Autodesk Fusion 360 part; units mm, degrees
(part 2 of 3)
sketch "Pocket SRL sketch" plane through (0, 0, 0) normal (0, 0, 1) x (1, 0, 0) in component "Upper frame"
  line L0 (-81.4, 57.15) -> (-81.4, 62.85)
  line L1 (-81.4, 62.85) -> (-62.2, 62.85)
  line L2 (-62.2, 62.85) -> (-62.2, 57.15)
  line L3 (-62.2, 57.15) -> (-81.4, 57.15)
extrude "Pocket SRL" cut sketch "Pocket SRL sketch" along normal blind 24 from surface at 89 bodies 27 in component "Upper frame"
sketch "Beam SRL sketch" plane through (0, 0, 0) normal (0, 0, 1) x (1, 0, 0) in component "Upper frame"
  line L0 (-80.8, 60) -> (-80.8, 80.6769)
  line L1 (-80.8, 80.6769) -> (-62.8, 80.6769)
  line L2 (-62.8, 80.6769) -> (-62.8, 60)
  line L3 (-62.8, 60) -> (-80.8, 60)
extrude "Beam SRL" cut sketch "Beam SRL sketch" along normal blind 18 from surface at 91 bodies 27 in component "Upper frame"
sketch "Pocket SRR sketch" plane through (0, 0, 0) normal (0, 0, 1) x (1, 0, 0) in component "Upper frame"
  line L0 (-62.2, -57.15) -> (-62.2, -62.85)
  line L1 (-62.2, -62.85) -> (-81.4, -62.85)
  line L2 (-81.4, -62.85) -> (-81.4, -57.15)
  line L3 (-81.4, -57.15) -> (-62.2, -57.15)
extrude "Pocket SRR" cut sketch "Pocket SRR sketch" along normal blind 24 from surface at 89 bodies 27 in component "Upper frame"
sketch "Beam SRR sketch" plane through (0, 0, 0) normal (0, 0, 1) x (1, 0, 0) in component "Upper frame"
  line L0 (-62.8, -60) -> (-62.8, -80.6769)
  line L1 (-62.8, -80.6769) -> (-80.8, -80.6769)
  line L2 (-80.8, -80.6769) -> (-80.8, -60)
  line L3 (-80.8, -60) -> (-62.8, -60)
extrude "Beam SRR" cut sketch "Beam SRR sketch" along normal blind 18 from surface at 91 bodies 27 in component "Upper frame"
sketch "Pocket RL sketch" plane through (0, 0, 0) normal (0, 0, 1) x (1, 0, 0) in component "Upper frame"
  line L0 (-81.15, 35.4) -> (-86.85, 35.4)
  line L1 (-86.85, 35.4) -> (-86.85, 54.6)
  line L2 (-86.85, 54.6) -> (-81.15, 54.6)
  line L3 (-81.15, 54.6) -> (-81.15, 35.4)
extrude "Pocket RL" cut sketch "Pocket RL sketch" along normal blind 24 from surface at 89 bodies 27 in component "Upper frame"
sketch "Beam RL sketch" plane through (0, 0, 0) normal (0, 0, 1) x (1, 0, 0) in component "Upper frame"
  line L0 (-84, 36) -> (-98.1784, 36)
  line L1 (-98.1784, 36) -> (-98.1784, 54)
  line L2 (-98.1784, 54) -> (-84, 54)
  line L3 (-84, 54) -> (-84, 36)
extrude "Beam RL" cut sketch "Beam RL sketch" along normal blind 18 from surface at 91 bodies 27 in component "Upper frame"
sketch "Pocket RR sketch" plane through (0, 0, 0) normal (0, 0, 1) x (1, 0, 0) in component "Upper frame"
  line L0 (-81.15, -54.6) -> (-86.85, -54.6)
  line L1 (-86.85, -54.6) -> (-86.85, -35.4)
  line L2 (-86.85, -35.4) -> (-81.15, -35.4)
  line L3 (-81.15, -35.4) -> (-81.15, -54.6)
extrude "Pocket RR" cut sketch "Pocket RR sketch" along normal blind 24 from surface at 89 bodies 27 in component "Upper frame"
sketch "Beam RR sketch" plane through (0, 0, 0) normal (0, 0, 1) x (1, 0, 0) in component "Upper frame"
  line L0 (-84, -54) -> (-98.1784, -54)
  line L1 (-98.1784, -54) -> (-98.1784, -36)
  line L2 (-98.1784, -36) -> (-84, -36)
  line L3 (-84, -36) -> (-84, -54)
extrude "Beam RR" cut sketch "Beam RR sketch" along normal blind 18 from surface at 91 bodies 27 in component "Upper frame"
sketch "Camera window L sketch" plane through (0, 0, 0) normal (0, 1, 0) x (1, 0, 0) in component "Upper frame"
  line L0 (-10.9288, -86) -> (17.0712, -86)
  line L1 (17.0712, -86) -> (17.0712, -106)
  line L2 (17.0712, -106) -> (-10.9288, -106)
  line L3 (-10.9288, -106) -> (-10.9288, -86)
extrude "Camera window L" cut sketch "Camera window L sketch" along normal blind 24 from surface at 84 bodies 27 in component "Upper frame"
sketch "Camera window R sketch" plane through (0, 0, 0) normal (0, 1, 0) x (1, 0, 0) in component "Upper frame"
  line L0 (-10.9288, -86) -> (17.0712, -86)
  line L1 (17.0712, -86) -> (17.0712, -106)
  line L2 (17.0712, -106) -> (-10.9288, -106)
  line L3 (-10.9288, -106) -> (-10.9288, -86)
extrude "Camera window R" cut sketch "Camera window R sketch" along normal blind 24 from surface at -108 bodies 27 in component "Upper frame"
sketch "VL53L0X module F sketch" plane through (0, 0, 0) normal (0, 0, 1) x (1, 0, 0) in component "ToF F"
  line L0 (92.75, -9) -> (97.25, -9)
  line L1 (97.25, -9) -> (97.25, 9)
  line L2 (97.25, 9) -> (92.75, 9)
  line L3 (92.75, 9) -> (92.75, -9)
extrude "VL53L0X module F" add sketch "VL53L0X module F sketch" along normal blind 21 from surface at 89.5 separate body makes body 28 in component "ToF F"
sketch "VL53L0X chip F sketch" plane through (0, 0, 0) normal (0, 0, 1) x (1, 0, 0) in component "ToF F"
  line L0 (97.25, -2.2) -> (98.25, -2.2)
  line L1 (98.25, -2.2) -> (98.25, 2.2)
  line L2 (98.25, 2.2) -> (97.25, 2.2)
  line L3 (97.25, 2.2) -> (97.25, -2.2)
extrude "VL53L0X chip F" add sketch "VL53L0X chip F sketch" along normal blind 2.4 from surface at 98.8 separate body makes body 29 in component "ToF F"
sketch "VL53L0X module FL sketch" plane through (0, 0, 0) normal (0, 0, 1) x (1, 0, 0) in component "ToF FL"
  line L0 (91.4888, 32.7315) -> (95.5672, 34.6333)
  line L1 (95.5672, 34.6333) -> (87.9601, 50.9469)
  line L2 (87.9601, 50.9469) -> (83.8817, 49.0451)
  line L3 (83.8817, 49.0451) -> (91.4888, 32.7315)
extrude "VL53L0X module FL" add sketch "VL53L0X module FL sketch" along normal blind 21 from surface at 89.5 separate body makes body 30 in component "ToF FL"
sketch "VL53L0X chip FL sketch" plane through (0, 0, 0) normal (0, 0, 1) x (1, 0, 0) in component "ToF FL"
  line L0 (92.6934, 40.7962) -> (93.5997, 41.2188)
  line L1 (93.5997, 41.2188) -> (91.7402, 45.2066)
  line L2 (91.7402, 45.2066) -> (90.8339, 44.784)
  line L3 (90.8339, 44.784) -> (92.6934, 40.7962)
extrude "VL53L0X chip FL" add sketch "VL53L0X chip FL sketch" along normal blind 2.4 from surface at 98.8 separate body makes body 31 in component "ToF FL"
sketch "VL53L0X module FR sketch" plane through (0, 0, 0) normal (0, 0, 1) x (1, 0, 0) in component "ToF FR"
  line L0 (83.8817, -49.0451) -> (87.9601, -50.9469)
  line L1 (87.9601, -50.9469) -> (95.5672, -34.6333)
  line L2 (95.5672, -34.6333) -> (91.4888, -32.7315)
  line L3 (91.4888, -32.7315) -> (83.8817, -49.0451)
extrude "VL53L0X module FR" add sketch "VL53L0X module FR sketch" along normal blind 21 from surface at 89.5 separate body makes body 32 in component "ToF FR"
sketch "VL53L0X chip FR sketch" plane through (0, 0, 0) normal (0, 0, 1) x (1, 0, 0) in component "ToF FR"
  line L0 (90.8339, -44.784) -> (91.7402, -45.2066)
  line L1 (91.7402, -45.2066) -> (93.5997, -41.2188)
  line L2 (93.5997, -41.2188) -> (92.6934, -40.7962)
  line L3 (92.6934, -40.7962) -> (90.8339, -44.784)
extrude "VL53L0X chip FR" add sketch "VL53L0X chip FR sketch" along normal blind 2.4 from surface at 98.8 separate body makes body 33 in component "ToF FR"
sketch "VL53L0X module SFL sketch" plane through (0, 0, 0) normal (0, 0, 1) x (1, 0, 0) in component "ToF SFL"
  line L0 (80.8, 57.75) -> (80.8, 62.25)
  line L1 (80.8, 62.25) -> (62.8, 62.25)
  line L2 (62.8, 62.25) -> (62.8, 57.75)
  line L3 (62.8, 57.75) -> (80.8, 57.75)
extrude "VL53L0X module SFL" add sketch "VL53L0X module SFL sketch" along normal blind 21 from surface at 89.5 separate body makes body 34 in component "ToF SFL"
sketch "VL53L0X chip SFL sketch" plane through (0, 0, 0) normal (0, 0, 1) x (1, 0, 0) in component "ToF SFL"
  line L0 (74, 62.25) -> (74, 63.25)
  line L1 (74, 63.25) -> (69.6, 63.25)
  line L2 (69.6, 63.25) -> (69.6, 62.25)
  line L3 (69.6, 62.25) -> (74, 62.25)
extrude "VL53L0X chip SFL" add sketch "VL53L0X chip SFL sketch" along normal blind 2.4 from surface at 98.8 separate body makes body 35 in component "ToF SFL"
sketch "VL53L0X module SFR sketch" plane through (0, 0, 0) normal (0, 0, 1) x (1, 0, 0) in component "ToF SFR"
  line L0 (62.8, -57.75) -> (62.8, -62.25)
  line L1 (62.8, -62.25) -> (80.8, -62.25)
  line L2 (80.8, -62.25) -> (80.8, -57.75)
  line L3 (80.8, -57.75) -> (62.8, -57.75)
extrude "VL53L0X module SFR" add sketch "VL53L0X module SFR sketch" along normal blind 21 from surface at 89.5 separate body makes body 36 in component "ToF SFR"
sketch "VL53L0X chip SFR sketch" plane through (0, 0, 0) normal (0, 0, 1) x (1, 0, 0) in component "ToF SFR"
  line L0 (69.6, -62.25) -> (69.6, -63.25)
  line L1 (69.6, -63.25) -> (74, -63.25)
  line L2 (74, -63.25) -> (74, -62.25)
  line L3 (74, -62.25) -> (69.6, -62.25)
extrude "VL53L0X chip SFR" add sketch "VL53L0X chip SFR sketch" along normal blind 2.4 from surface at 98.8 separate body makes body 37 in component "ToF SFR"
sketch "VL53L0X module SRL sketch" plane through (0, 0, 0) normal (0, 0, 1) x (1, 0, 0) in component "ToF SRL"
  line L0 (-62.8, 57.75) -> (-62.8, 62.25)
  line L1 (-62.8, 62.25) -> (-80.8, 62.25)
  line L2 (-80.8, 62.25) -> (-80.8, 57.75)
  line L3 (-80.8, 57.75) -> (-62.8, 57.75)
extrude "VL53L0X module SRL" add sketch "VL53L0X module SRL sketch" along normal blind 21 from surface at 89.5 separate body makes body 38 in component "ToF SRL"
sketch "VL53L0X chip SRL sketch" plane through (0, 0, 0) normal (0, 0, 1) x (1, 0, 0) in component "ToF SRL"
  line L0 (-69.6, 62.25) -> (-69.6, 63.25)
  line L1 (-69.6, 63.25) -> (-74, 63.25)
  line L2 (-74, 63.25) -> (-74, 62.25)
  line L3 (-74, 62.25) -> (-69.6, 62.25)
extrude "VL53L0X chip SRL" add sketch "VL53L0X chip SRL sketch" along normal blind 2.4 from surface at 98.8 separate body makes body 39 in component "ToF SRL"
sketch "VL53L0X module SRR sketch" plane through (0, 0, 0) normal (0, 0, 1) x (1, 0, 0) in component "ToF SRR"
  line L0 (-80.8, -57.75) -> (-80.8, -62.25)
  line L1 (-80.8, -62.25) -> (-62.8, -62.25)
  line L2 (-62.8, -62.25) -> (-62.8, -57.75)
  line L3 (-62.8, -57.75) -> (-80.8, -57.75)
extrude "VL53L0X module SRR" add sketch "VL53L0X module SRR sketch" along normal blind 21 from surface at 89.5 separate body makes body 40 in component "ToF SRR"
sketch "VL53L0X chip SRR sketch" plane through (0, 0, 0) normal (0, 0, 1) x (1, 0, 0) in component "ToF SRR"
  line L0 (-74, -62.25) -> (-74, -63.25)
  line L1 (-74, -63.25) -> (-69.6, -63.25)
  line L2 (-69.6, -63.25) -> (-69.6, -62.25)
  line L3 (-69.6, -62.25) -> (-74, -62.25)
extrude "VL53L0X chip SRR" add sketch "VL53L0X chip SRR sketch" along normal blind 2.4 from surface at 98.8 separate body makes body 41 in component "ToF SRR"
sketch "VL53L0X module RL sketch" plane through (0, 0, 0) normal (0, 0, 1) x (1, 0, 0) in component "ToF RL"
  line L0 (-81.75, 54) -> (-86.25, 54)
  line L1 (-86.25, 54) -> (-86.25, 36)
  line L2 (-86.25, 36) -> (-81.75, 36)
  line L3 (-81.75, 36) -> (-81.75, 54)
extrude "VL53L0X module RL" add sketch "VL53L0X module RL sketch" along normal blind 21 from surface at 89.5 separate body makes body 42 in component "ToF RL"
sketch "VL53L0X chip RL sketch" plane through (0, 0, 0) normal (0, 0, 1) x (1, 0, 0) in component "ToF RL"
  line L0 (-86.25, 47.2) -> (-87.25, 47.2)
  line L1 (-87.25, 47.2) -> (-87.25, 42.8)
  line L2 (-87.25, 42.8) -> (-86.25, 42.8)
  line L3 (-86.25, 42.8) -> (-86.25, 47.2)
extrude "VL53L0X chip RL" add sketch "VL53L0X chip RL sketch" along normal blind 2.4 from surface at 98.8 separate body makes body 43 in component "ToF RL"
sketch "VL53L0X module RR sketch" plane through (0, 0, 0) normal (0, 0, 1) x (1, 0, 0) in component "ToF RR"
  line L0 (-81.75, -36) -> (-86.25, -36)
  line L1 (-86.25, -36) -> (-86.25, -54)
  line L2 (-86.25, -54) -> (-81.75, -54)
  line L3 (-81.75, -54) -> (-81.75, -36)
extrude "VL53L0X module RR" add sketch "VL53L0X module RR sketch" along normal blind 21 from surface at 89.5 separate body makes body 44 in component "ToF RR"
sketch "VL53L0X chip RR sketch" plane through (0, 0, 0) normal (0, 0, 1) x (1, 0, 0) in component "ToF RR"
  line L0 (-86.25, -42.8) -> (-87.25, -42.8)
  line L1 (-87.25, -42.8) -> (-87.25, -47.2)
  line L2 (-87.25, -47.2) -> (-86.25, -47.2)
  line L3 (-86.25, -47.2) -> (-86.25, -42.8)
extrude "VL53L0X chip RR" add sketch "VL53L0X chip RR sketch" along normal blind 2.4 from surface at 98.8 separate body makes body 45 in component "ToF RR"
sketch "Lens block L sketch" plane through (0, 0, 0) normal (0, 0, 1) x (1, 0, 0) in component "Camera L"
  line L0 (-10, -10) -> (10, -10)
  line L1 (10, -10) -> (10, 10)
  line L2 (10, 10) -> (-10, 10)
  line L3 (-10, 10) -> (-10, -10)
extrude "Lens block L" add sketch "Lens block L sketch" along normal blind 23 separate body makes body 46 in component "Camera L"
sketch "Lens holder L sketch" plane through (0, 0, 0) normal (0, 0, 1) x (1, 0, 0) in component "Camera L"
  line L0 (-10, -10) -> (10, -10)
  line L1 (10, -10) -> (10, 10)
  line L2 (10, 10) -> (-10, 10)
  line L3 (-10, 10) -> (-10, -10)
extrude "Lens holder L" add sketch "Lens holder L sketch" along normal blind 2 from surface at 23 bodies 46 in component "Camera L"
sketch "OpenMV H7 Plus board L sketch" plane through (0, 0, 0) normal (0, 0, 1) x (1, 0, 0) in component "Camera L"
  line L0 (-22.5, -18) -> (22.5, -18)
  line L1 (22.5, -18) -> (22.5, 18)
  line L2 (22.5, 18) -> (-22.5, 18)
  line L3 (-22.5, 18) -> (-22.5, -18)
extrude "OpenMV H7 Plus board L" add sketch "OpenMV H7 Plus board L sketch" along normal blind 6 from surface at 25 separate body makes body 47 in component "Camera L"
sketch "Lens block R sketch" plane through (0, 0, 0) normal (0, 0, 1) x (1, 0, 0) in component "Camera R"
  line L0 (-10, -10) -> (10, -10)
  line L1 (10, -10) -> (10, 10)
  line L2 (10, 10) -> (-10, 10)
  line L3 (-10, 10) -> (-10, -10)
extrude "Lens block R" add sketch "Lens block R sketch" along normal blind 23 separate body makes body 48 in component "Camera R"
sketch "Lens holder R sketch" plane through (0, 0, 0) normal (0, 0, 1) x (1, 0, 0) in component "Camera R"
  line L0 (-10, -10) -> (10, -10)
  line L1 (10, -10) -> (10, 10)
  line L2 (10, 10) -> (-10, 10)
  line L3 (-10, 10) -> (-10, -10)
extrude "Lens holder R" add sketch "Lens holder R sketch" along normal blind 2 from surface at 23 bodies 48 in component "Camera R"
sketch "OpenMV H7 Plus board R sketch" plane through (0, 0, 0) normal (0, 0, 1) x (1, 0, 0) in component "Camera R"
  line L0 (-22.5, -18) -> (22.5, -18)
  line L1 (22.5, -18) -> (22.5, 18)
  line L2 (22.5, 18) -> (-22.5, 18)
  line L3 (-22.5, 18) -> (-22.5, -18)
extrude "OpenMV H7 Plus board R" add sketch "OpenMV H7 Plus board R sketch" along normal blind 6 from surface at 25 separate body makes body 49 in component "Camera R"
sketch "Lid plate sketch" plane through (0, 0, 0) normal (0, 0, 1) x (1, 0, 0) in component "Lid"
  circle A0 centre (0, 0) radius 105
extrude "Lid plate" add sketch "Lid plate sketch" along normal blind 3 from surface at 112 separate body makes body 50 in component "Lid"
sketch "Camera hump sketch" plane through (0, 0, 0) normal (0, 0, 1) x (1, 0, 0) in component "Lid"
  line L0 (-21.9288, 53) -> (28.0712, 53)
  line L1 (28.0712, 53) -> (28.0712, 93)
  line L2 (28.0712, 93) -> (-21.9288, 93)
  line L3 (-21.9288, 93) -> (-21.9288, 53)
extrude "Camera hump" add sketch "Camera hump sketch" along normal blind 8.5 from surface at 114.5 bodies 50 in component "Lid"
sketch "Camera hump sketch (1)" plane through (0, 0, 0) normal (0, 0, 1) x (1, 0, 0) in component "Lid"
  line L0 (-21.9288, -93) -> (28.0712, -93)
  line L1 (28.0712, -93) -> (28.0712, -53)
  line L2 (28.0712, -53) -> (-21.9288, -53)
  line L3 (-21.9288, -53) -> (-21.9288, -93)
extrude "Camera hump (1)" add sketch "Camera hump sketch (1)" along normal blind 8.5 from surface at 114.5 bodies 50 in component "Lid"
sketch "Camera pocket sketch" plane through (0, 0, 0) normal (0, 0, 1) x (1, 0, 0) in component "Lid"
  line L0 (-19.9288, 55) -> (26.0712, 55)
  line L1 (26.0712, 55) -> (26.0712, 91)
  line L2 (26.0712, 91) -> (-19.9288, 91)
  line L3 (-19.9288, 91) -> (-19.9288, 55)
extrude "Camera pocket" cut sketch "Camera pocket sketch" along normal blind 10 from surface at 111 bodies 50 in component "Lid"
sketch "Camera pocket sketch (1)" plane through (0, 0, 0) normal (0, 0, 1) x (1, 0, 0) in component "Lid"
  line L0 (-19.9288, -91) -> (26.0712, -91)
  line L1 (26.0712, -91) -> (26.0712, -55)
  line L2 (26.0712, -55) -> (-19.9288, -55)
  line L3 (-19.9288, -55) -> (-19.9288, -91)
extrude "Camera pocket (1)" cut sketch "Camera pocket sketch (1)" along normal blind 10 from surface at 111 bodies 50 in component "Lid"
sketch "Handle slot sketch" plane through (0, 0, 0) normal (0, 0, 1) x (1, 0, 0) in component "Lid"
  line L0 (29.5, -9) -> (90.5, -9)
  line L1 (90.5, -9) -> (90.5, 9)
  line L2 (90.5, 9) -> (29.5, 9)
  line L3 (29.5, 9) -> (29.5, -9)
extrude "Handle slot" cut sketch "Handle slot sketch" along normal blind 5 from surface at 111 bodies 50 in component "Lid"
sketch "Front notch sketch" plane through (0, 0, 0) normal (0, 0, 1) x (1, 0, 0) in component "Lid"
  line L0 (49, 7) -> (92, 7)
  line L1 (92, 7) -> (92, 35)
  line L2 (92, 35) -> (49, 35)
  line L3 (49, 35) -> (49, 7)
extrude "Front notch" cut sketch "Front notch sketch" along normal blind 5 from surface at 111 bodies 50 in component "Lid"
sketch "Finger notch sketch" plane through (0, 0, 0) normal (0, 0, 1) x (1, 0, 0) in component "Lid"
  line L0 (97.4603, 17.6488) -> (105.2855, 19.3121)
  line L1 (105.2855, 19.3121) -> (104.0381, 25.181)
  line L2 (104.0381, 25.181) -> (96.2129, 23.5177)
  line L3 (96.2129, 23.5177) -> (97.4603, 17.6488)
extrude "Finger notch" cut sketch "Finger notch sketch" along normal blind 5 from surface at 111 bodies 50 in component "Lid"
sketch "Finger notch sketch (1)" plane through (0, 0, 0) normal (0, 0, 1) x (1, 0, 0) in component "Lid"
  line L0 (96.2129, -23.5177) -> (104.0381, -25.181)
  line L1 (104.0381, -25.181) -> (105.2855, -19.3121)
  line L2 (105.2855, -19.3121) -> (97.4603, -17.6488)
  line L3 (97.4603, -17.6488) -> (96.2129, -23.5177)
extrude "Finger notch (1)" cut sketch "Finger notch sketch (1)" along normal blind 5 from surface at 111 bodies 50 in component "Lid"
sketch "Hook skirt +71 sketch" plane through (0, 0, 0) normal (0, 0, 1) x (1, 0, 0) in component "Lid"
  arc A0 (43.5428, 95.5459) -> (24.5118, 102.0988) centre (0, 0) ccw
  line L0 (24.5118, 102.0988) -> (24.1383, 100.543)
  arc A1 (42.8793, 94.09) -> (24.1383, 100.543) centre (0, 0) ccw
  line L1 (42.8793, 94.09) -> (43.5428, 95.5459)
extrude "Hook skirt +71" add sketch "Hook skirt +71 sketch" along normal blind 8.5 from surface at 104 bodies 50 in component "Lid"
sketch "Hook bump +71 sketch" plane through (0, 0, 0) normal (0, 0, 1) x (1, 0, 0) in component "Lid"
  arc A0 (41.3104, 95.0074) -> (25.9394, 100.3001) centre (0, 0) ccw
  line L0 (25.9394, 100.3001) -> (25.6389, 99.1383)
  arc A1 (40.8319, 93.907) -> (25.6389, 99.1383) centre (0, 0) ccw
  line L1 (40.8319, 93.907) -> (41.3104, 95.0074)
extrude "Hook bump +71" add sketch "Hook bump +71 sketch" along normal blind 3 from surface at 105.5 separate body makes body 51 in component "Lid"
sketch "Hook skirt +114 sketch" plane through (0, 0, 0) normal (0, 0, 1) x (1, 0, 0) in component "Lid"
  arc A0 (-33.317, 99.574) -> (-51.7045, 91.3873) centre (0, 0) ccw
  line L0 (-51.7045, 91.3873) -> (-50.9166, 89.9948)
  arc A1 (-32.8093, 98.0567) -> (-50.9166, 89.9948) centre (0, 0) ccw
  line L1 (-32.8093, 98.0567) -> (-33.317, 99.574)
extrude "Hook skirt +114" add sketch "Hook skirt +114 sketch" along normal blind 8.5 from surface at 104 bodies 50 in component "Lid"
sketch "Hook bump +114 sketch" plane through (0, 0, 0) normal (0, 0, 1) x (1, 0, 0) in component "Lid"
  arc A0 (-34.5824, 97.6577) -> (-49.4336, 91.0455) centre (0, 0) ccw
  line L0 (-49.4336, 91.0455) -> (-48.8611, 89.9909)
  arc A1 (-34.1818, 96.5265) -> (-48.8611, 89.9909) centre (0, 0) ccw
  line L1 (-34.1818, 96.5265) -> (-34.5824, 97.6577)
extrude "Hook bump +114" add sketch "Hook bump +114 sketch" along normal blind 3 from surface at 105.5 separate body makes body 52 in component "Lid"
sketch "Hook skirt -71 sketch" plane through (0, 0, 0) normal (0, 0, 1) x (1, 0, 0) in component "Lid"
  arc A0 (24.5118, -102.0988) -> (43.5428, -95.5459) centre (0, 0) ccw
  line L0 (43.5428, -95.5459) -> (42.8793, -94.09)
  arc A1 (24.1383, -100.543) -> (42.8793, -94.09) centre (0, 0) ccw
  line L1 (24.1383, -100.543) -> (24.5118, -102.0988)
extrude "Hook skirt -71" add sketch "Hook skirt -71 sketch" along normal blind 8.5 from surface at 104 bodies 50 in component "Lid"
sketch "Hook bump -71 sketch" plane through (0, 0, 0) normal (0, 0, 1) x (1, 0, 0) in component "Lid"
  arc A0 (25.9394, -100.3001) -> (41.3104, -95.0074) centre (0, 0) ccw
  line L0 (41.3104, -95.0074) -> (40.8319, -93.907)
  arc A1 (25.6389, -99.1383) -> (40.8319, -93.907) centre (0, 0) ccw
  line L1 (25.6389, -99.1383) -> (25.9394, -100.3001)
extrude "Hook bump -71" add sketch "Hook bump -71 sketch" along normal blind 3 from surface at 105.5 separate body makes body 53 in component "Lid"
sketch "Hook skirt -114 sketch" plane through (0, 0, 0) normal (0, 0, 1) x (1, 0, 0) in component "Lid"
  arc A0 (-51.7045, -91.3873) -> (-33.317, -99.574) centre (0, 0) ccw
  line L0 (-33.317, -99.574) -> (-32.8093, -98.0567)
  arc A1 (-50.9166, -89.9948) -> (-32.8093, -98.0567) centre (0, 0) ccw
  line L1 (-50.9166, -89.9948) -> (-51.7045, -91.3873)
extrude "Hook skirt -114" add sketch "Hook skirt -114 sketch" along normal blind 8.5 from surface at 104 bodies 50 in component "Lid"
sketch "Hook bump -114 sketch" plane through (0, 0, 0) normal (0, 0, 1) x (1, 0, 0) in component "Lid"
  arc A0 (-49.4336, -91.0455) -> (-34.5824, -97.6577) centre (0, 0) ccw
  line L0 (-34.5824, -97.6577) -> (-34.1818, -96.5265)
  arc A1 (-48.8611, -89.9909) -> (-34.1818, -96.5265) centre (0, 0) ccw
  line L1 (-48.8611, -89.9909) -> (-49.4336, -91.0455)
extrude "Hook bump -114" add sketch "Hook bump -114 sketch" along normal blind 3 from surface at 105.5 separate body makes body 54 in component "Lid"
sketch "Handle bar sketch" plane through (0, 0, 0) normal (0, 0, 1) x (1, 0, 0) in component "Handle bar"
  line L0 (33, -8) -> (87, -8)
  line L1 (87, -8) -> (87, 8)
  line L2 (87, 8) -> (33, 8)
  line L3 (33, 8) -> (33, -8)
extrude "Handle bar" add sketch "Handle bar sketch" along normal blind 16 from surface at 140 separate body makes body 55 in component "Handle bar"
sketch "Victim LED sketch" plane through (0, 0, 0) normal (0, 0, 1) x (1, 0, 0) in component "Victim LED"
  circle A0 centre (83.5, 0) radius 2.5
extrude "Victim LED" add sketch "Victim LED sketch" along normal blind 4 from surface at 156 separate body makes body 56 in component "Victim LED"
sketch "Start button sketch" plane through (0, 0, 0) normal (0, 0, 1) x (1, 0, 0) in component "Start button"
  circle A0 centre (75.5, 21.5) radius 6
extrude "Start button" add sketch "Start button sketch" along normal blind 7 from surface at 90 separate body makes body 57 in component "Start button"
sketch "Power switch sketch" plane through (0, 0, 0) normal (0, 0, 1) x (1, 0, 0) in component "Power switch"
  line L0 (53.5, 12) -> (66.5, 12)
  line L1 (66.5, 12) -> (66.5, 31)
  line L2 (66.5, 31) -> (53.5, 31)
  line L3 (53.5, 31) -> (53.5, 12)
extrude "Power switch" add sketch "Power switch sketch" along normal blind 13 from surface at 90 separate body makes body 58 in component "Power switch"
sketch "Status LED 1 sketch" plane through (0, 0, 0) normal (0, 0, 1) x (1, 0, 0) in component "Status LED 1"
  circle A0 centre (75, 0) radius 2
extrude "Status LED 1" add sketch "Status LED 1 sketch" along normal blind 4 from surface at 98 separate body makes body 59 in component "Status LED 1"
sketch "Status LED 2 sketch" plane through (0, 0, 0) normal (0, 0, 1) x (1, 0, 0) in component "Status LED 2"
  circle A0 centre (66, 0) radius 2
extrude "Status LED 2" add sketch "Status LED 2 sketch" along normal blind 4 from surface at 98 separate body makes body 60 in component "Status LED 2"
sketch "USB-C service socket sketch" plane through (0, 0, 0) normal (0, 0, 1) x (1, 0, 0) in component "USB-C service socket"
  line L0 (80.9456, -43.1544) -> (92.8217, -48.442)
  line L1 (92.8217, -48.442) -> (98.1093, -36.5659)
  line L2 (98.1093, -36.5659) -> (86.2332, -31.2784)
  line L3 (86.2332, -31.2784) -> (80.9456, -43.1544)
extrude "USB-C service socket" add sketch "USB-C service socket sketch" along normal blind 7 from surface at 71.5 separate body makes body 61 in component "USB-C service socket"
sketch "Dropper floor sketch" plane through (0, 0, 0) normal (0, 0, 1) x (1, 0, 0) in component "Dropper floor"
  circle A0 centre (-20, 0) radius 51.1342
extrude "Dropper floor" add sketch "Dropper floor sketch" along normal blind 3 from surface at 87 separate body makes body 62 in component "Dropper floor"
sketch "Dropper floor tab 0 sketch" plane through (0, 0, 0) normal (0, 0, 1) x (1, 0, 0) in component "Dropper floor"
  line L0 (30, 8.5) -> (39, 8.5)
  line L1 (39, 8.5) -> (39, 12.5)
  line L2 (39, 12.5) -> (30, 12.5)
  line L3 (30, 12.5) -> (30, 8.5)
extrude "Dropper floor tab 0" add sketch "Dropper floor tab 0 sketch" along normal blind 1.5 from surface at 88.5 bodies 62 in component "Dropper floor"
sketch "Dropper floor tab 1 sketch" plane through (0, 0, 0) normal (0, 0, 1) x (1, 0, 0) in component "Dropper floor"
  line L0 (30, -12.5) -> (39, -12.5)
  line L1 (39, -12.5) -> (39, -8.5)
  line L2 (39, -8.5) -> (30, -8.5)
  line L3 (30, -8.5) -> (30, -12.5)
extrude "Dropper floor tab 1" add sketch "Dropper floor tab 1 sketch" along normal blind 1.5 from surface at 88.5 bodies 62 in component "Dropper floor"
sketch "Dropper floor tab 2 sketch" plane through (0, 0, 0) normal (0, 0, 1) x (1, 0, 0) in component "Dropper floor"
  line L0 (-75, -5) -> (-69, -5)
  line L1 (-69, -5) -> (-69, 5)
  line L2 (-69, 5) -> (-75, 5)
  line L3 (-75, 5) -> (-75, -5)
extrude "Dropper floor tab 2" add sketch "Dropper floor tab 2 sketch" along normal blind 1.5 from surface at 88.5 bodies 62 in component "Dropper floor"
sketch "Slot A sketch" plane through (0, 0, 0) normal (0, 0, 1) x (1, 0, 0) in component "Dropper floor"
  line L0 (-47.2943, -37.5474) -> (-37.0413, -27.2943)
  line L1 (-37.0413, -27.2943) -> (-47.2943, -17.0413)
  line L2 (-47.2943, -17.0413) -> (-57.5474, -27.2943)
  line L3 (-57.5474, -27.2943) -> (-47.2943, -37.5474)
extrude "Slot A" cut sketch "Slot A sketch" along normal blind 5 from surface at 86 bodies 62 in component "Dropper floor"
sketch "Slot B sketch" plane through (0, 0, 0) normal (0, 0, 1) x (1, 0, 0) in component "Dropper floor"
  line L0 (-47.2943, 17.0413) -> (-37.0413, 27.2943)
  line L1 (-37.0413, 27.2943) -> (-47.2943, 37.5474)
  line L2 (-47.2943, 37.5474) -> (-57.5474, 27.2943)
  line L3 (-57.5474, 27.2943) -> (-47.2943, 17.0413)
extrude "Slot B" cut sketch "Slot B sketch" along normal blind 5 from surface at 86 bodies 62 in component "Dropper floor"
sketch "N20 pocket sketch" plane through (0, 0, 0) normal (0, 0, 1) x (1, 0, 0) in component "Dropper floor"
  line L0 (-25.2, -6.2) -> (-14.8, -6.2)
  line L1 (-14.8, -6.2) -> (-14.8, 6.2)
  line L2 (-14.8, 6.2) -> (-25.2, 6.2)
  line L3 (-25.2, 6.2) -> (-25.2, -6.2)
extrude "N20 pocket" cut sketch "N20 pocket sketch" along normal blind 5 from surface at 86 bodies 62 in component "Dropper floor"
sketch "N20 face plate recess sketch" plane through (0, 0, 0) normal (0, 0, 1) x (1, 0, 0) in component "Dropper floor"
  line L0 (-28.2, -9.2) -> (-11.8, -9.2)
  line L1 (-11.8, -9.2) -> (-11.8, 9.2)
  line L2 (-11.8, 9.2) -> (-28.2, 9.2)
  line L3 (-28.2, 9.2) -> (-28.2, -9.2)
extrude "N20 face plate recess" cut sketch "N20 face plate recess sketch" along normal blind 3 from surface at 88 bodies 62 in component "Dropper floor"
sketch "Dropper plate sketch" plane through (0, 0, 0) normal (0, 0, 1) x (1, 0, 0) in component "Dropper plate"
  circle A0 centre (-20, 0) radius 49.1342
extrude "Dropper plate" add sketch "Dropper plate sketch" along normal blind 12 from surface at 90 separate body makes body 63 in component "Dropper plate"
sketch "Pocket 1 sketch" plane through (0, 0, 0) normal (0, 0, 1) x (1, 0, 0) in component "Dropper plate"
  line L0 (-34.9402, -28.7115) -> (-38.5636, -42.2345)
  line L1 (-38.5636, -42.2345) -> (-25.0407, -45.858)
  line L2 (-25.0407, -45.858) -> (-21.4172, -32.335)
  line L3 (-21.4172, -32.335) -> (-34.9402, -28.7115)
extrude "Pocket 1" cut sketch "Pocket 1 sketch" along normal blind 14 from surface at 89 bodies 63 in component "Dropper plate"
sketch "Pocket 2 sketch" plane through (0, 0, 0) normal (0, 0, 1) x (1, 0, 0) in component "Dropper plate"
  line L0 (-18.5828, -32.335) -> (-14.9593, -45.858)
  line L1 (-14.9593, -45.858) -> (-1.4364, -42.2345)
  line L2 (-1.4364, -42.2345) -> (-5.0598, -28.7115)
  line L3 (-5.0598, -28.7115) -> (-18.5828, -32.335)
extrude "Pocket 2" cut sketch "Pocket 2 sketch" along normal blind 14 from surface at 89 bodies 63 in component "Dropper plate"
sketch "Pocket 3 sketch" plane through (0, 0, 0) normal (0, 0, 1) x (1, 0, 0) in component "Dropper plate"
  line L0 (-2.6052, -27.2943) -> (7.2943, -37.1938)
  line L1 (7.2943, -37.1938) -> (17.1938, -27.2943)
  line L2 (17.1938, -27.2943) -> (7.2943, -17.3948)
  line L3 (7.2943, -17.3948) -> (-2.6052, -27.2943)
extrude "Pocket 3" cut sketch "Pocket 3 sketch" along normal blind 14 from surface at 89 bodies 63 in component "Dropper plate"
sketch "Pocket 4 sketch" plane through (0, 0, 0) normal (0, 0, 1) x (1, 0, 0) in component "Dropper plate"
  line L0 (8.7115, -14.9402) -> (22.2345, -18.5636)
  line L1 (22.2345, -18.5636) -> (25.858, -5.0407)
  line L2 (25.858, -5.0407) -> (12.335, -1.4172)
  line L3 (12.335, -1.4172) -> (8.7115, -14.9402)
extrude "Pocket 4" cut sketch "Pocket 4 sketch" along normal blind 14 from surface at 89 bodies 63 in component "Dropper plate"
sketch "Pocket 5 sketch" plane through (0, 0, 0) normal (0, 0, 1) x (1, 0, 0) in component "Dropper plate"
  line L0 (12.335, 1.4172) -> (25.858, 5.0407)
  line L1 (25.858, 5.0407) -> (22.2345, 18.5636)
  line L2 (22.2345, 18.5636) -> (8.7115, 14.9402)
  line L3 (8.7115, 14.9402) -> (12.335, 1.4172)
extrude "Pocket 5" cut sketch "Pocket 5 sketch" along normal blind 14 from surface at 89 bodies 63 in component "Dropper plate"
sketch "Pocket 6 sketch" plane through (0, 0, 0) normal (0, 0, 1) x (1, 0, 0) in component "Dropper plate"
  line L0 (7.2943, 17.3948) -> (17.1938, 27.2943)
  line L1 (17.1938, 27.2943) -> (7.2943, 37.1938)
  line L2 (7.2943, 37.1938) -> (-2.6052, 27.2943)
  line L3 (-2.6052, 27.2943) -> (7.2943, 17.3948)
extrude "Pocket 6" cut sketch "Pocket 6 sketch" along normal blind 14 from surface at 89 bodies 63 in component "Dropper plate"
sketch "Pocket 7 sketch" plane through (0, 0, 0) normal (0, 0, 1) x (1, 0, 0) in component "Dropper plate"
  line L0 (-5.0598, 28.7115) -> (-1.4364, 42.2345)
  line L1 (-1.4364, 42.2345) -> (-14.9593, 45.858)
  line L2 (-14.9593, 45.858) -> (-18.5828, 32.335)
  line L3 (-18.5828, 32.335) -> (-5.0598, 28.7115)
extrude "Pocket 7" cut sketch "Pocket 7 sketch" along normal blind 14 from surface at 89 bodies 63 in component "Dropper plate"
sketch "Pocket 8 sketch" plane through (0, 0, 0) normal (0, 0, 1) x (1, 0, 0) in component "Dropper plate"
  line L0 (-21.4172, 32.335) -> (-25.0407, 45.858)
  line L1 (-25.0407, 45.858) -> (-38.5636, 42.2345)
  line L2 (-38.5636, 42.2345) -> (-34.9402, 28.7115)
  line L3 (-34.9402, 28.7115) -> (-21.4172, 32.335)
extrude "Pocket 8" cut sketch "Pocket 8 sketch" along normal blind 14 from surface at 89 bodies 63 in component "Dropper plate"
sketch "Shaft bore sketch (5)" plane through (0, 0, 0) normal (0, 0, 1) x (1, 0, 0) in component "Dropper plate"
  circle A0 centre (-20, 0) radius 1.5
extrude "Shaft bore''''" cut sketch "Shaft bore sketch (5)" along normal blind 14 from surface at 89 bodies 63 in component "Dropper plate"
sketch "N20 gearmotor with encoder sketch" plane through (0, 0, 0) normal (0, 0, 1) x (1, 0, 0) in component "N20 motor"
  line L0 (-25, -6) -> (-15, -6)
  line L1 (-15, -6) -> (-15, 6)
  line L2 (-15, 6) -> (-25, 6)
  line L3 (-25, 6) -> (-25, -6)
extrude "N20 gearmotor with encoder" add sketch "N20 gearmotor with encoder sketch" along normal blind 41.5 from surface at 46.5 separate body makes body 64 in component "N20 motor"
sketch "N20 shaft sketch" plane through (0, 0, 0) normal (0, 0, 1) x (1, 0, 0) in component "N20 motor"
  circle A0 centre (-20, 0) radius 1.5
extrude "N20 shaft" add sketch "N20 shaft sketch" along normal blind 10 from surface at 88 separate body makes body 65 in component "N20 motor"
sketch "N20 face plate sketch" plane through (0, 0, 0) normal (0, 0, 1) x (1, 0, 0) in component "N20 face plate"
  line L0 (-28, -9) -> (-12, -9)
  line L1 (-12, -9) -> (-12, 9)
  line L2 (-12, 9) -> (-28, 9)
  line L3 (-28, 9) -> (-28, -9)
extrude "N20 face plate" add sketch "N20 face plate sketch" along normal blind 2 from surface at 88 separate body makes body 66 in component "N20 face plate"
sketch "Shaft bore sketch (6)" plane through (0, 0, 0) normal (0, 0, 1) x (1, 0, 0) in component "N20 face plate"
  circle A0 centre (-20, 0) radius 1.7
extrude "Shaft bore'''''" cut sketch "Shaft bore sketch (6)" along normal blind 4 from surface at 87 bodies 66 in component "N20 face plate"
sketch "Kit 1 sketch" plane through (0, 0, 0) normal (0, 0, 1) x (1, 0, 0) in component "Kits"
  line L0 (-33.632, -30.9773) -> (-36.2979, -40.9263)
  line L1 (-36.2979, -40.9263) -> (-26.3488, -43.5922)
  line L2 (-26.3488, -43.5922) -> (-23.683, -33.6431)
  line L3 (-23.683, -33.6431) -> (-33.632, -30.9773)
extrude "Kit 1" add sketch "Kit 1 sketch" along normal blind 10.3 from surface at 90 separate body makes body 67 in component "Kits"
sketch "Kit 2 sketch" plane through (0, 0, 0) normal (0, 0, 1) x (1, 0, 0) in component "Kits"
  line L0 (-16.317, -33.6431) -> (-13.6512, -43.5922)
  line L1 (-13.6512, -43.5922) -> (-3.7021, -40.9263)
  line L2 (-3.7021, -40.9263) -> (-6.368, -30.9773)
  line L3 (-6.368, -30.9773) -> (-16.317, -33.6431)
extrude "Kit 2" add sketch "Kit 2 sketch" along normal blind 10.3 from surface at 90 separate body makes body 68 in component "Kits"
sketch "Kit 3 sketch" plane through (0, 0, 0) normal (0, 0, 1) x (1, 0, 0) in component "Kits"
  line L0 (0.0111, -27.2943) -> (7.2943, -34.5775)
  line L1 (7.2943, -34.5775) -> (14.5775, -27.2943)
  line L2 (14.5775, -27.2943) -> (7.2943, -20.0111)
  line L3 (7.2943, -20.0111) -> (0.0111, -27.2943)
extrude "Kit 3" add sketch "Kit 3 sketch" along normal blind 10.3 from surface at 90 separate body makes body 69 in component "Kits"
sketch "Kit 4 sketch" plane through (0, 0, 0) normal (0, 0, 1) x (1, 0, 0) in component "Kits"
  line L0 (10.9773, -13.632) -> (20.9263, -16.2979)
  line L1 (20.9263, -16.2979) -> (23.5922, -6.3488)
  line L2 (23.5922, -6.3488) -> (13.6431, -3.683)
  line L3 (13.6431, -3.683) -> (10.9773, -13.632)
extrude "Kit 4" add sketch "Kit 4 sketch" along normal blind 10.3 from surface at 90 separate body makes body 70 in component "Kits"
sketch "Kit 5 sketch" plane through (0, 0, 0) normal (0, 0, 1) x (1, 0, 0) in component "Kits"
  line L0 (13.6431, 3.683) -> (23.5922, 6.3488)
  line L1 (23.5922, 6.3488) -> (20.9263, 16.2979)
  line L2 (20.9263, 16.2979) -> (10.9773, 13.632)
  line L3 (10.9773, 13.632) -> (13.6431, 3.683)
extrude "Kit 5" add sketch "Kit 5 sketch" along normal blind 10.3 from surface at 90 separate body makes body 71 in component "Kits"
sketch "Kit 6 sketch" plane through (0, 0, 0) normal (0, 0, 1) x (1, 0, 0) in component "Kits"
  line L0 (7.2943, 20.0111) -> (14.5775, 27.2943)
  line L1 (14.5775, 27.2943) -> (7.2943, 34.5775)
  line L2 (7.2943, 34.5775) -> (0.0111, 27.2943)
  line L3 (0.0111, 27.2943) -> (7.2943, 20.0111)
extrude "Kit 6" add sketch "Kit 6 sketch" along normal blind 10.3 from surface at 90 separate body makes body 72 in component "Kits"
sketch "Kit 7 sketch" plane through (0, 0, 0) normal (0, 0, 1) x (1, 0, 0) in component "Kits"
  line L0 (-6.368, 30.9773) -> (-3.7021, 40.9263)
  line L1 (-3.7021, 40.9263) -> (-13.6512, 43.5922)
  line L2 (-13.6512, 43.5922) -> (-16.317, 33.6431)
  line L3 (-16.317, 33.6431) -> (-6.368, 30.9773)
extrude "Kit 7" add sketch "Kit 7 sketch" along normal blind 10.3 from surface at 90 separate body makes body 73 in component "Kits"
sketch "Kit 8 sketch" plane through (0, 0, 0) normal (0, 0, 1) x (1, 0, 0) in component "Kits"
  line L0 (-23.683, 33.6431) -> (-26.3488, 43.5922)
  line L1 (-26.3488, 43.5922) -> (-36.2979, 40.9263)
  line L2 (-36.2979, 40.9263) -> (-33.632, 30.9773)
  line L3 (-33.632, 30.9773) -> (-23.683, 33.6431)
extrude "Kit 8" add sketch "Kit 8 sketch" along normal blind 10.3 from surface at 90 separate body makes body 74 in component "Kits"
sketch "Hopper sketch" plane through (0, 0, 0) normal (0, 0, 1) x (1, 0, 0) in component "Hopper B left"
  line L0 (-47.2943, 13.5057) -> (-33.5057, 27.2943)
  line L1 (-33.5057, 27.2943) -> (-47.2943, 41.0829)
  line L2 (-47.2943, 41.0829) -> (-61.0829, 27.2943)
  line L3 (-61.0829, 27.2943) -> (-47.2943, 13.5057)
extrude "Hopper" add sketch "Hopper sketch" along normal blind 15 from surface at 72 separate body makes body 75 in component "Hopper B left"
sketch "Hopper flange sketch" plane through (0, 0, 0) normal (0, 0, 1) x (1, 0, 0) in component "Hopper B left"
  line L0 (-47.2943, 10.6773) -> (-30.6773, 27.2943)
  line L1 (-30.6773, 27.2943) -> (-47.2943, 43.9113)
  line L2 (-47.2943, 43.9113) -> (-63.9113, 27.2943)
  line L3 (-63.9113, 27.2943) -> (-47.2943, 10.6773)
extrude "Hopper flange" add sketch "Hopper flange sketch" along normal blind 1.5 from surface at 85.5 bodies 75 in component "Hopper B left"
sketch "Hopper void sketch" plane through (0, 0, 0) normal (0, 0, 1) x (1, 0, 0) in component "Hopper B left"
  line L0 (-47.2943, 17.0413) -> (-37.0413, 27.2943)
  line L1 (-37.0413, 27.2943) -> (-47.2943, 37.5474)
  line L2 (-47.2943, 37.5474) -> (-57.5474, 27.2943)
  line L3 (-57.5474, 27.2943) -> (-47.2943, 17.0413)
extrude "Hopper void" cut sketch "Hopper void sketch" along normal blind 14.4 from surface at 73.6 bodies 75 in component "Hopper B left"
sketch "Socket tool sketch" plane through (0, 0, 0) normal (0, 0, 1) x (1, 0, 0) in component "Hopper B left"
  line L0 (-8.1, -8.1) -> (8.1, -8.1)
  line L1 (8.1, -8.1) -> (8.1, 8.1)
  line L2 (8.1, 8.1) -> (-8.1, 8.1)
  line L3 (-8.1, 8.1) -> (-8.1, -8.1)
extrude "Socket tool" add sketch "Socket tool sketch" along normal blind 35 separate body makes body 76 in component "Hopper B left"
move_body "Move1'" bodies 76 to x (-0.977496, -0.210954, 0) y (-0.112564, 0.521586, 0.845741) z (-0.178413, 0.826708, -0.533594) at (-46.4023, 23.1608, 82.168) in component "Hopper B left"
combine "Combine1'" operation cut target body 75 tool bodies 76 in component "Hopper B left"
sketch "Channel sketch" plane through (0, 0, 0) normal (0, 0, 1) x (1, 0, 0) in component "Chute B left"
  line L0 (-8.1, -8.1) -> (8.1, -8.1)
  line L1 (8.1, -8.1) -> (8.1, 8.1)
  line L2 (8.1, 8.1) -> (-8.1, 8.1)
  line L3 (-8.1, 8.1) -> (-8.1, -8.1)
extrude "Channel" add sketch "Channel sketch" along normal blind 79.2151 separate body makes body 77 in component "Chute B left"
move_body "Move1''" bodies 77 to x (-0.977496, -0.210954, 0) y (-0.112564, 0.521586, 0.845741) z (-0.178413, 0.826708, -0.533594) at (-47.2943, 27.2943, 79.5) in component "Chute B left"
sketch "Channel void sketch" plane through (0, 0, 0) normal (0, 0, 1) x (1, 0, 0) in component "Chute B left"
  line L0 (-6.5, -6.5) -> (6.5, -6.5)
  line L1 (6.5, -6.5) -> (6.5, 6.5)
  line L2 (6.5, 6.5) -> (-6.5, 6.5)
  line L3 (-6.5, 6.5) -> (-6.5, -6.5)
extrude "Channel void" add sketch "Channel void sketch" along normal blind 83.2151 separate body makes body 78 in component "Chute B left"
move_body "Move2'" bodies 78 to x (-0.977496, -0.210954, 0) y (-0.112564, 0.521586, 0.845741) z (-0.178413, 0.826708, -0.533594) at (-46.9375, 25.6409, 80.5672) in component "Chute B left"
combine "Combine1''" operation cut target body 77 tool bodies 78 in component "Chute B left"
sketch "Trough cut sketch" plane through (0, 0, 0) normal (0, 0, 1) x (1, 0, 0) in component "Chute B left"
  line L0 (-47.2943, 17.0413) -> (-37.0413, 27.2943)
  line L1 (-37.0413, 27.2943) -> (-47.2943, 37.5474)
  line L2 (-47.2943, 37.5474) -> (-57.5474, 27.2943)
  line L3 (-57.5474, 27.2943) -> (-47.2943, 17.0413)
extrude "Trough cut" cut sketch "Trough cut sketch" along normal blind 13 from surface at 77 bodies 77 in component "Chute B left"
sketch "Trim sketch" plane through (0, 0, 0) normal (0, 0, 1) x (1, 0, 0) in component "Chute B left"
  circle A0 centre (0, 0) radius 140
  circle A1 centre (0, 0) radius 105
extrude "Trim" add sketch "Trim sketch" along normal blind 70 from surface at 20 separate body makes body 79 in component "Chute B left"
combine "Combine2'" operation cut target body 77 tool bodies 79 in component "Chute B left"
sketch "Hopper sketch (2)" plane through (0, 0, 0) normal (0, 0, 1) x (1, 0, 0) in component "Hopper A right"
  line L0 (-47.2943, -41.0829) -> (-33.5057, -27.2943)
  line L1 (-33.5057, -27.2943) -> (-47.2943, -13.5057)
  line L2 (-47.2943, -13.5057) -> (-61.0829, -27.2943)
  line L3 (-61.0829, -27.2943) -> (-47.2943, -41.0829)
extrude "Hopper'" add sketch "Hopper sketch (2)" along normal blind 15 from surface at 72 separate body makes body 80 in component "Hopper A right"
sketch "Hopper flange sketch (2)" plane through (0, 0, 0) normal (0, 0, 1) x (1, 0, 0) in component "Hopper A right"
  line L0 (-47.2943, -43.9113) -> (-30.6773, -27.2943)
  line L1 (-30.6773, -27.2943) -> (-47.2943, -10.6773)
  line L2 (-47.2943, -10.6773) -> (-63.9113, -27.2943)
  line L3 (-63.9113, -27.2943) -> (-47.2943, -43.9113)
extrude "Hopper flange'" add sketch "Hopper flange sketch (2)" along normal blind 1.5 from surface at 85.5 bodies 80 in component "Hopper A right"
sketch "Hopper void sketch (2)" plane through (0, 0, 0) normal (0, 0, 1) x (1, 0, 0) in component "Hopper A right"
  line L0 (-47.2943, -37.5474) -> (-37.0413, -27.2943)
  line L1 (-37.0413, -27.2943) -> (-47.2943, -17.0413)
  line L2 (-47.2943, -17.0413) -> (-57.5474, -27.2943)
  line L3 (-57.5474, -27.2943) -> (-47.2943, -37.5474)
extrude "Hopper void'" cut sketch "Hopper void sketch (2)" along normal blind 14.4 from surface at 73.6 bodies 80 in component "Hopper A right"
sketch "Socket tool sketch (2)" plane through (0, 0, 0) normal (0, 0, 1) x (1, 0, 0) in component "Hopper A right"
  line L0 (-8.1, -8.1) -> (8.1, -8.1)
  line L1 (8.1, -8.1) -> (8.1, 8.1)
  line L2 (8.1, 8.1) -> (-8.1, 8.1)
  line L3 (-8.1, 8.1) -> (-8.1, -8.1)
extrude "Socket tool'" add sketch "Socket tool sketch (2)" along normal blind 35 separate body makes body 81 in component "Hopper A right"
move_body "Move1'''" bodies 81 to x (0.977496, -0.210954, 0) y (-0.112564, -0.521586, 0.845741) z (-0.178413, -0.826708, -0.533594) at (-46.4023, -23.1608, 82.168) in component "Hopper A right"
combine "Combine1'''" operation cut target body 80 tool bodies 81 in component "Hopper A right"
sketch "Channel sketch (2)" plane through (0, 0, 0) normal (0, 0, 1) x (1, 0, 0) in component "Chute A right"
  line L0 (-8.1, -8.1) -> (8.1, -8.1)
  line L1 (8.1, -8.1) -> (8.1, 8.1)
  line L2 (8.1, 8.1) -> (-8.1, 8.1)
  line L3 (-8.1, 8.1) -> (-8.1, -8.1)
extrude "Channel'" add sketch "Channel sketch (2)" along normal blind 79.2151 separate body makes body 82 in component "Chute A right"
move_body "Move1''''" bodies 82 to x (0.977496, -0.210954, 0) y (-0.112564, -0.521586, 0.845741) z (-0.178413, -0.826708, -0.533594) at (-47.2943, -27.2943, 79.5) in component "Chute A right"
sketch "Channel void sketch (2)" plane through (0, 0, 0) normal (0, 0, 1) x (1, 0, 0) in component "Chute A right"
  line L0 (-6.5, -6.5) -> (6.5, -6.5)
  line L1 (6.5, -6.5) -> (6.5, 6.5)
  line L2 (6.5, 6.5) -> (-6.5, 6.5)
  line L3 (-6.5, 6.5) -> (-6.5, -6.5)
extrude "Channel void'" add sketch "Channel void sketch (2)" along normal blind 83.2151 separate body makes body 83 in component "Chute A right"
move_body "Move2''" bodies 83 to x (0.977496, -0.210954, 0) y (-0.112564, -0.521586, 0.845741) z (-0.178413, -0.826708, -0.533594) at (-46.9375, -25.6409, 80.5672) in component "Chute A right"
combine "Combine1''''" operation cut target body 82 tool bodies 83 in component "Chute A right"
sketch "Trough cut sketch (2)" plane through (0, 0, 0) normal (0, 0, 1) x (1, 0, 0) in component "Chute A right"
  line L0 (-47.2943, -37.5474) -> (-37.0413, -27.2943)
  line L1 (-37.0413, -27.2943) -> (-47.2943, -17.0413)
  line L2 (-47.2943, -17.0413) -> (-57.5474, -27.2943)
  line L3 (-57.5474, -27.2943) -> (-47.2943, -37.5474)
extrude "Trough cut'" cut sketch "Trough cut sketch (2)" along normal blind 13 from surface at 77 bodies 82 in component "Chute A right"
sketch "Trim sketch (2)" plane through (0, 0, 0) normal (0, 0, 1) x (1, 0, 0) in component "Chute A right"
  circle A0 centre (0, 0) radius 140
  circle A1 centre (0, 0) radius 105
extrude "Trim'" add sketch "Trim sketch (2)" along normal blind 70 from surface at 20 separate body makes body 84 in component "Chute A right"
combine "Combine2''" operation cut target body 82 tool bodies 84 in component "Chute A right"
sketch "GIGA post H1 sketch" plane through (0, 0, 0) normal (0, 0, 1) x (1, 0, 0) in component "GIGA posts"
  circle A0 centre (58.72, -16.17) radius 3.5
extrude "GIGA post H1" add sketch "GIGA post H1 sketch" along normal blind 22.5 from surface at 39 separate body makes body 85 in component "GIGA posts"
sketch "Insert hole H1 sketch" plane through (0, 0, 0) normal (0, 0, 1) x (1, 0, 0) in component "GIGA posts"
  circle A0 centre (58.72, -16.17) radius 2
extrude "Insert hole H1" cut sketch "Insert hole H1 sketch" along normal blind 7 from surface at 55.5 bodies 85 in component "GIGA posts"
sketch "GIGA post H2 sketch" plane through (0, 0, 0) normal (0, 0, 1) x (1, 0, 0) in component "GIGA posts"
  circle A0 centre (-16.21, -16.17) radius 3.5
extrude "GIGA post H2" add sketch "GIGA post H2 sketch" along normal blind 22.5 from surface at 39 separate body makes body 86 in component "GIGA posts"
sketch "Insert hole H2 sketch" plane through (0, 0, 0) normal (0, 0, 1) x (1, 0, 0) in component "GIGA posts"
  circle A0 centre (-16.21, -16.17) radius 2
extrude "Insert hole H2" cut sketch "Insert hole H2 sketch" along normal blind 7 from surface at 55.5 bodies 86 in component "GIGA posts"
sketch "GIGA post H3 sketch" plane through (0, 0, 0) normal (0, 0, 1) x (1, 0, 0) in component "GIGA posts"
  circle A0 centre (60.06, -64.33) radius 3.5
extrude "GIGA post H3" add sketch "GIGA post H3 sketch" along normal blind 22.5 from surface at 39 separate body makes body 87 in component "GIGA posts"
sketch "Insert hole H3 sketch" plane through (0, 0, 0) normal (0, 0, 1) x (1, 0, 0) in component "GIGA posts"
  circle A0 centre (60.06, -64.33) radius 2
extrude "Insert hole H3" cut sketch "Insert hole H3 sketch" along normal blind 7 from surface at 55.5 bodies 87 in component "GIGA posts"
sketch "GIGA post H4 sketch" plane through (0, 0, 0) normal (0, 0, 1) x (1, 0, 0) in component "GIGA posts"
  circle A0 centre (-22.74, -64.33) radius 3.5
extrude "GIGA post H4" add sketch "GIGA post H4 sketch" along normal blind 22.5 from surface at 39 separate body makes body 88 in component "GIGA posts"
sketch "Insert hole H4 sketch" plane through (0, 0, 0) normal (0, 0, 1) x (1, 0, 0) in component "GIGA posts"
  circle A0 centre (-22.74, -64.33) radius 2
extrude "Insert hole H4" cut sketch "Insert hole H4 sketch" along normal blind 7 from surface at 55.5 bodies 88 in component "GIGA posts"
sketch "GIGA board sketch" plane through (0, 0, 0) normal (0, 0, 1) x (1, 0, 0) in component "Arduino GIGA R1"
  line L0 (-27.56, -66.97) -> (73.96, -66.97)
  line L1 (73.96, -66.97) -> (73.96, -13.63)
  line L2 (73.96, -13.63) -> (-27.56, -13.63)
  line L3 (-27.56, -13.63) -> (-27.56, -66.97)
extrude "GIGA board" add sketch "GIGA board sketch" along normal blind 1.6 from surface at 61.5 separate body makes body 89 in component "Arduino GIGA R1"
sketch "Header strip +y sketch" plane through (0, 0, 0) normal (0, 0, 1) x (1, 0, 0) in component "Arduino GIGA R1"
  line L0 (-23.56, -17.38) -> (69.96, -17.38)
  line L1 (69.96, -17.38) -> (69.96, -14.88)
  line L2 (69.96, -14.88) -> (-23.56, -14.88)
  line L3 (-23.56, -14.88) -> (-23.56, -17.38)
extrude "Header strip +y" add sketch "Header strip +y sketch" along normal blind 8.5 from surface at 63.1 separate body makes body 90 in component "Arduino GIGA R1"
sketch "Header strip -y sketch" plane through (0, 0, 0) normal (0, 0, 1) x (1, 0, 0) in component "Arduino GIGA R1"
  line L0 (-23.56, -65.72) -> (69.96, -65.72)
  line L1 (69.96, -65.72) -> (69.96, -63.22)
  line L2 (69.96, -63.22) -> (-23.56, -63.22)
  line L3 (-23.56, -63.22) -> (-23.56, -65.72)
extrude "Header strip -y" add sketch "Header strip -y sketch" along normal blind 8.5 from surface at 63.1 separate body makes body 91 in component "Arduino GIGA R1"
sketch "Main PCB shield (placeholder) sketch" plane through (0, 0, 0) normal (0, 0, 1) x (1, 0, 0) in component "Main PCB"
  line L0 (-27.56, -66.97) -> (73.96, -66.97)
  line L1 (73.96, -66.97) -> (73.96, -13.63)
  line L2 (73.96, -13.63) -> (-27.56, -13.63)
  line L3 (-27.56, -13.63) -> (-27.56, -66.97)
extrude "Main PCB shield (placeholder)" add sketch "Main PCB shield (placeholder) sketch" along normal blind 1.6 from surface at 71.6 separate body makes body 92 in component "Main PCB"
sketch "PCB component envelope (placeholder) sketch" plane through (0, 0, 0) normal (0, 0, 1) x (1, 0, 0) in component "Main PCB"
  line L0 (-24.56, -63.97) -> (70.96, -63.97)
  line L1 (70.96, -63.97) -> (70.96, -16.63)
  line L2 (70.96, -16.63) -> (-24.56, -16.63)
  line L3 (-24.56, -16.63) -> (-24.56, -63.97)
extrude "PCB component envelope (placeholder)" add sketch "PCB component envelope (placeholder) sketch" along normal blind 7.3 from surface at 73.2 separate body makes body 93 in component "Main PCB"